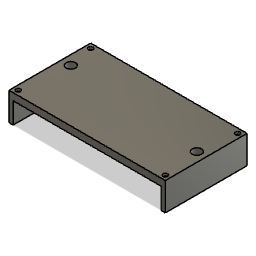
Device (Autodesk Fusion 360 archive; units mm, degrees)
design "button_holder"
Autodesk Fusion 360 part; units mm, degrees
(part 1 of 3)
sketch "Sketch1" plane through (0, 0, 0) normal (0, 1, 0) x (1, 0, 0)
  line L0 (33.5, 17.5) -> (-33.5, 17.5)
  line L1 (-33.5, 17.5) -> (-33.5, -17.5)
  line L2 (-33.5, -17.5) -> (33.5, -17.5)
  line L3 (33.5, -17.5) -> (33.5, 17.5)
  line L4 (33.5, 17.5) -> (-33.5, -17.5) construction
  line L5 (-33.5, 17.5) -> (33.5, -17.5) construction
  dimension "d1" = 67
  dimension "d2" = 35
  constraint horizontal L0
  constraint perpendicular L0 L1
  constraint parallel L0 L2
  constraint parallel L1 L3
  constraint coincident L4 origin
  constraint coincident L5 origin
  measures "d1" distance of L1.end L2.end
  measures "d2" distance of L0.end L1.end
extrude "Extrude1" add sketch "Sketch1" along normal blind 3
sketch "Sketch2" plane through (0, 0, 0) normal (0, -1, 0) x (1, 0, 0)
  line L0 (33.5, -17.5) -> (33.5, 17.5)
  line L1 (33.5, 17.5) -> (-33.5, 17.5)
  line L2 (-33.5, 17.5) -> (-33.5, -17.5)
  line L3 (-33.5, -17.5) -> (33.5, -17.5)
  line L4 (-33.5, 17.5) -> (-31.7, 17.5)
  line L5 (-31.7, 17.5) -> (-31.7, -17.5)
  line L6 (-31.7, -17.5) -> (-33.5, -17.5)
  line L7 (-33.5, -17.5) -> (-33.5, 17.5)
  line L8 (33.5, 17.5) -> (31.7, 17.5)
  line L9 (31.7, 17.5) -> (31.7, -17.5)
  line L10 (31.7, -17.5) -> (33.5, -17.5)
  line L11 (33.5, -17.5) -> (33.5, 17.5)
  dimension "d5" = 1.8
  dimension "d6" = 35
  dimension "d7" = 1.8
  dimension "d8" = 35
  constraint horizontal L4
  constraint vertical L5
  constraint horizontal L6
  constraint vertical L7
  constraint coincident L1.end L2.start
  constraint horizontal L8
  constraint vertical L9
  constraint horizontal L10
  constraint vertical L11
  constraint coincident L0.end L1.start
  measures "d5" distance of L1.end L4.end
  measures "d6" distance of L1.end L2.end
  measures "d7" distance of L0.end L8.end
  measures "d8" distance of L0.end L0.start
extrude "Extrude2" add sketch "Sketch2" along normal blind 9 contours L0 L1 L3 L8 L9 L10 L11 | L1 L2 L3 L4 L5 L6 L7
sketch "Sketch3" plane through (0, 3, 0) normal (0, 1, 0) x (-1, 0, 0)
  line L0 (-33.5, 17.5) -> (-33.5, -17.5)
  line L1 (-33.5, -17.5) -> (33.5, -17.5)
  line L2 (33.5, -17.5) -> (33.5, 17.5)
  line L3 (33.5, 17.5) -> (-33.5, 17.5)
  line L4 (33.5, -17.5) -> (31.5, -17.5)
  line L5 (31.5, -17.5) -> (31.5, -15.5)
  line L6 (31.5, -15.5) -> (33.5, -15.5)
  line L7 (33.5, -15.5) -> (33.5, -17.5)
  line L8 (33.5, 17.5) -> (31.5, 17.5)
  line L9 (31.5, 17.5) -> (31.5, 15.5)
  line L10 (31.5, 15.5) -> (33.5, 15.5)
  line L11 (33.5, 15.5) -> (33.5, 17.5)
  line L12 (-33.5, -17.5) -> (-31.5, -17.5)
  line L13 (-31.5, -17.5) -> (-31.5, -15.5)
  line L14 (-31.5, -15.5) -> (-33.5, -15.5)
  line L15 (-33.5, -15.5) -> (-33.5, -17.5)
  line L16 (-33.5, 17.5) -> (-31.5, 17.5)
  line L17 (-31.5, 17.5) -> (-31.5, 15.5)
  line L18 (-31.5, 15.5) -> (-33.5, 15.5)
  line L19 (-33.5, 15.5) -> (-33.5, 17.5)
  circle A0 centre (-31.5, 15.5) radius 1
  circle A1 centre (-31.5, -15.5) radius 1
  circle A2 centre (31.5, -15.5) radius 1
  circle A3 centre (31.5, 15.5) radius 1
  dimension "d11" = 2
  dimension "d12" = 2
  dimension "d13" = 2
  dimension "d14" = 2
  dimension "d15" = 2
  dimension "d16" = 2
  dimension "d17" = 2
  dimension "d18" = 2
  dimension "d19" = 2
  dimension "d20" = 2
  dimension "d21" = 2
  dimension "d24" = 2
  constraint horizontal L4
  constraint vertical L5
  constraint horizontal L6
  constraint vertical L7
  constraint coincident L1.end L2.start
  constraint horizontal L8
  constraint vertical L9
  constraint horizontal L10
  constraint vertical L11
  constraint coincident L2.end L3.start
  constraint horizontal L12
  constraint vertical L13
  constraint horizontal L14
  constraint vertical L15
  constraint coincident L0.end L1.start
  constraint horizontal L16
  constraint vertical L17
  constraint horizontal L18
  constraint vertical L19
  constraint coincident L0.start L3.end
  constraint coincident L17.end L18.start
  constraint coincident L13.end L14.start
  constraint coincident L5.end L6.start
  constraint coincident L9.end L10.start
  measures "d11" distance of L1.end L4.end
  measures "d12" distance of L2.end L8.end
  measures "d13" distance of L2.end L10.end
  measures "d14" distance of L0.end L12.end
  measures "d15" distance of L0.end L14.end
  measures "d16" distance of L0.start L16.end
  measures "d17" distance of L0.start L18.end
  measures "d18" diameter of A0
  measures "d19" diameter of A1
  measures "d20" diameter of A2
  measures "d21" diameter of A3
  measures "d24" distance of L1.end L6.end
extrude "Extrude3" cut sketch "Sketch3" against normal blind 1 contours L17 L18 A0 | L17 L18 A0 | L13 L14 A1 | L13 L14 A1 | L9 L10 A3 | L9 L10 A3 | L5 L6 A2 | L5 L6 A2
sketch "Sketch4" plane through (0, 3, 0) normal (0, 1, 0) x (-1, 0, 0)
  circle A0 centre (31.5, -15.5) radius 1
  circle A1 centre (-31.5, -15.5) radius 1
  circle A2 centre (31.5, 15.5) radius 1
  circle A3 centre (-31.5, 15.5) radius 1
  line L0 (-33.5, 17.5) -> (-33.5, -17.5)
  line L1 (-33.5, -17.5) -> (33.5, -17.5)
  line L2 (33.5, -17.5) -> (33.5, 17.5)
  line L3 (33.5, 17.5) -> (-33.5, 17.5)
  line L4 (-33.5, 0) -> (-29.5, 0)
  line L5 (-29.5, 0) -> (-29.5, -1)
  line L6 (-29.5, -1) -> (-33.5, -1)
  line L7 (-33.5, -1) -> (-33.5, 0)
  circle A4 centre (-29.5, 0) radius 2
  line L8 (33.5, 0) -> (29.5, 0)
  line L9 (29.5, 0) -> (29.5, -5)
  line L10 (29.5, -5) -> (33.5, -5)
  line L11 (33.5, -5) -> (33.5, 0)
  circle A5 centre (29.5, -5) radius 2
  dimension "d27" = 4
  dimension "d28" = 1
  dimension "d29" = 4
  dimension "d33" = 4
  dimension "d34" = 5
  dimension "d35" = 4
  constraint horizontal L4
  constraint vertical L5
  constraint horizontal L6
  constraint vertical L7
  constraint midpoint L0 L4.start
  constraint coincident L4.end L5.start
  constraint horizontal L8
  constraint vertical L9
  constraint horizontal L10
  constraint vertical L11
  constraint midpoint L2 L8.start
  constraint coincident L9.end L10.start
  measures "d27" distance of L4.start L4.end
  measures "d28" distance of L4.start L6.end
  measures "d29" diameter of A4
  measures "d33" distance of L8.start L8.end
  measures "d34" distance of L8.start L10.end
  measures "d35" diameter of A5
extrude "Extrude4" cut sketch "Sketch4" against normal blind 5 contours L4 L5 L6 A4 | L4 L5 L6 A4 | L9 L10 A5 | L9 L10 A5

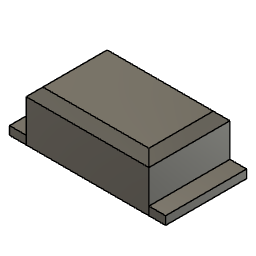
design "klavesa"
Autodesk Fusion 360 part; units mm, degrees
sketch "Sketch1" plane through (0, 0, 0) normal (0, 1, 0) x (1, 0, 0)
  line L0 (7.35, 4.85) -> (-7.35, 4.85)
  line L1 (-7.35, 4.85) -> (-7.35, -4.85)
  line L2 (-7.35, -4.85) -> (7.35, -4.85)
  line L3 (7.35, -4.85) -> (7.35, 4.85)
  line L4 (7.35, 4.85) -> (-7.35, -4.85) construction
  line L5 (-7.35, 4.85) -> (7.35, -4.85) construction
  line L6 (-7.35, 4.85) -> (-9.35, 4.85)
  line L7 (-9.35, 4.85) -> (-9.35, -4.85)
  line L8 (-9.35, -4.85) -> (-7.35, -4.85)
  line L9 (-7.35, -4.85) -> (-7.35, 4.85)
  line L10 (7.35, 4.85) -> (9.35, 4.85)
  line L11 (9.35, 4.85) -> (9.35, -4.85)
  line L12 (9.35, -4.85) -> (7.35, -4.85)
  line L13 (7.35, -4.85) -> (7.35, 4.85)
  dimension "d1" = 14.7
  dimension "d2" = 9.7
  dimension "d10" = 2
  dimension "d11" = 9.7
  dimension "d12" = 2
  dimension "d13" = 9.7
  constraint horizontal L0
  constraint perpendicular L0 L1
  constraint parallel L0 L2
  constraint parallel L1 L3
  constraint coincident L4 origin
  constraint coincident L5 origin
  constraint horizontal L6
  constraint vertical L7
  constraint horizontal L8
  constraint vertical L9
  constraint horizontal L10
  constraint vertical L11
  constraint horizontal L12
  constraint vertical L13
  measures "d1" distance of L1.end L2.end
  measures "d2" distance of L0.end L1.end
  measures "d10" distance of L0.end L6.end
  measures "d11" distance of L0.end L1.end
  measures "d12" distance of L0.start L10.end
  measures "d13" distance of L0.start L2.end
extrude "Extrude3" add sketch "Sketch1" along normal blind 1 contours L3 L10 L11 L12 L13 | L1 L6 L7 L8 L9 makes body 1 at (8.6833, 0, 1.6167) makes body 2 at (-8.0167, 0, -1.6167)
extrude "Extrude1" add sketch "Sketch1" along normal blind 6 separate body contours L0 L1 L2 L3 L9 L13 makes body 3
chamfer "Chamfer1" distance 1 angle 45 4 edges at (0, 6, 4.85) (7.35, 6, 0) (-7.35, 6, 0) (0, 6, -4.85) measured on face at (-2.45, 6, 1.6167) measured on face at (-2.45, 6, 1.6167) measured on face at (-2.45, 6, 1.6167) measured on face at (-2.45, 6, 1.6167) on bodies 3
sketch "Sketch2" plane through (0, 0, 0) normal (0, -1, 0) x (1, 0, 0)
  line L0 (7.35, -4.85) -> (7.35, 4.85)
  line L1 (7.35, 4.85) -> (-7.35, 4.85)
  line L2 (-7.35, 4.85) -> (-7.35, -4.85)
  line L3 (-7.35, -4.85) -> (7.35, -4.85)
  circle A0 centre (0, 0) radius 1.7
  dimension "d7" = 3.4
  constraint coincident A0.centre origin
  measures "d7" diameter of A0
extrude "Extrude2" cut sketch "Sketch2" against normal blind 4 contours A0 bodies 3

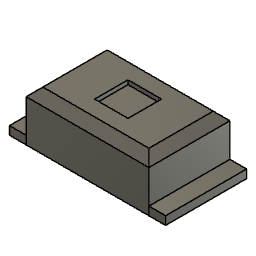
design "klavesa_stop"
Autodesk Fusion 360 part; units mm, degrees
sketch "Sketch1" plane through (0, 0, 0) normal (0, 1, 0) x (1, 0, 0)
  line L0 (7.35, 4.85) -> (-7.35, 4.85)
  line L1 (-7.35, 4.85) -> (-7.35, -4.85)
  line L2 (-7.35, -4.85) -> (7.35, -4.85)
  line L3 (7.35, -4.85) -> (7.35, 4.85)
  line L4 (7.35, 4.85) -> (-7.35, -4.85) construction
  line L5 (-7.35, 4.85) -> (7.35, -4.85) construction
  line L6 (-7.35, 4.85) -> (-9.35, 4.85)
  line L7 (-9.35, 4.85) -> (-9.35, -4.85)
  line L8 (-9.35, -4.85) -> (-7.35, -4.85)
  line L9 (-7.35, -4.85) -> (-7.35, 4.85)
  line L10 (7.35, 4.85) -> (9.35, 4.85)
  line L11 (9.35, 4.85) -> (9.35, -4.85)
  line L12 (9.35, -4.85) -> (7.35, -4.85)
  line L13 (7.35, -4.85) -> (7.35, 4.85)
  dimension "d1" = 14.7
  dimension "d2" = 9.7
  dimension "d10" = 2
  dimension "d11" = 9.7
  dimension "d12" = 2
  dimension "d13" = 9.7
  constraint horizontal L0
  constraint perpendicular L0 L1
  constraint parallel L0 L2
  constraint parallel L1 L3
  constraint coincident L4 origin
  constraint coincident L5 origin
  constraint horizontal L6
  constraint vertical L7
  constraint horizontal L8
  constraint vertical L9
  constraint horizontal L10
  constraint vertical L11
  constraint horizontal L12
  constraint vertical L13
  measures "d1" distance of L1.end L2.end
  measures "d2" distance of L0.end L1.end
  measures "d10" distance of L0.end L6.end
  measures "d11" distance of L0.end L1.end
  measures "d12" distance of L0.start L10.end
  measures "d13" distance of L0.start L2.end
extrude "Extrude3" add sketch "Sketch1" along normal blind 1 contours L3 L10 L11 L12 L13 | L1 L6 L7 L8 L9 makes body 1 at (8.6833, 0, 1.6167) makes body 2 at (-8.0167, 0, -1.6167)
extrude "Extrude1" add sketch "Sketch1" along normal blind 6 separate body contours L0 L1 L2 L3 L9 L13 makes body 3
chamfer "Chamfer1" distance 1 angle 45 4 edges at (0, 6, 4.85) (7.35, 6, 0) (-7.35, 6, 0) (0, 6, -4.85) measured on face at (-2.45, 6, 1.6167) measured on face at (-2.45, 6, 1.6167) measured on face at (-2.45, 6, 1.6167) measured on face at (-2.45, 6, 1.6167) on bodies 3
sketch "Sketch2" plane through (0, 0, 0) normal (0, -1, 0) x (1, 0, 0)
  line L0 (7.35, -4.85) -> (7.35, 4.85)
  line L1 (7.35, 4.85) -> (-7.35, 4.85)
  line L2 (-7.35, 4.85) -> (-7.35, -4.85)
  line L3 (-7.35, -4.85) -> (7.35, -4.85)
  circle A0 centre (0, 0) radius 1.7
  dimension "d7" = 3.4
  constraint coincident A0.centre origin
  measures "d7" diameter of A0
extrude "Extrude2" cut sketch "Sketch2" against normal blind 4 contours A0 bodies 3
sketch "Sketch3" plane through (0, 6, 0) normal (0, 1, 0) x (-1, 0, 0)
  line L0 (-6.35, -3.85) -> (6.35, -3.85)
  line L1 (6.35, -3.85) -> (6.35, 3.85)
  line L2 (6.35, 3.85) -> (-6.35, 3.85)
  line L3 (-6.35, 3.85) -> (-6.35, -3.85)
  line L4 (-2, -2) -> (2, -2)
  line L5 (2, -2) -> (2, 2)
  line L6 (2, 2) -> (-2, 2)
  line L7 (-2, 2) -> (-2, -2)
  line L8 (-2, -2) -> (2, 2) construction
  line L9 (2, -2) -> (-2, 2) construction
  dimension "d16" = 4
  dimension "d17" = 4
  constraint horizontal L4
  constraint perpendicular L4 L5
  constraint parallel L4 L6
  constraint parallel L5 L7
  constraint coincident L8 origin
  constraint coincident L9 origin
  measures "d16" distance of L5.end L6.end
  measures "d17" distance of L4.end L5.end
extrude "Extrude4" cut sketch "Sketch3" against normal blind 0.5 contours L4 L5 L6 L7 bodies 3

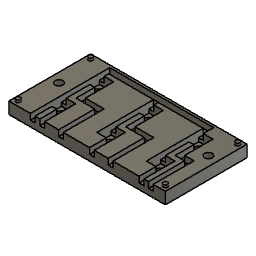
design "key_holder"
Autodesk Fusion 360 part; units mm, degrees
sketch "Sketch1" plane through (0, 0, 0) normal (0, 1, 0) x (1, 0, 0)
  line L0 (33.5, 17.5) -> (-33.5, 17.5)
  line L1 (-33.5, 17.5) -> (-33.5, -17.5)
  line L2 (-33.5, -17.5) -> (33.5, -17.5)
  line L3 (33.5, -17.5) -> (33.5, 17.5)
  line L4 (33.5, 17.5) -> (-33.5, -17.5) construction
  line L5 (-33.5, 17.5) -> (33.5, -17.5) construction
  dimension "d1" = 67
  dimension "d2" = 35
  constraint horizontal L0
  constraint perpendicular L0 L1
  constraint parallel L0 L2
  constraint parallel L1 L3
  constraint coincident L4 origin
  constraint coincident L5 origin
  measures "d1" distance of L1.end L2.end
  measures "d2" distance of L0.end L1.end
extrude "Extrude1" add sketch "Sketch1" along normal blind 5
sketch "Sketch2" plane through (0, 5, 0) normal (0, 1, 0) x (-1, 0, 0)
  line L0 (-33.5, 17.5) -> (-33.5, -17.5)
  line L1 (-33.5, -17.5) -> (33.5, -17.5)
  line L2 (33.5, -17.5) -> (33.5, 17.5)
  line L3 (33.5, 17.5) -> (-33.5, 17.5)
  line L4 (33.5, -17.5) -> (31.5, -17.5)
  line L5 (31.5, -17.5) -> (31.5, -15.5)
  line L6 (31.5, -15.5) -> (33.5, -15.5)
  line L7 (33.5, -15.5) -> (33.5, -17.5)
  line L8 (-33.5, -17.5) -> (-31.5, -17.5)
  line L9 (-31.5, -17.5) -> (-31.5, -15.5)
  line L10 (-31.5, -15.5) -> (-33.5, -15.5)
  line L11 (-33.5, -15.5) -> (-33.5, -17.5)
  line L12 (33.5, 17.5) -> (31.5, 17.5)
  line L13 (31.5, 17.5) -> (31.5, 15.5)
  line L14 (31.5, 15.5) -> (33.5, 15.5)
  line L15 (33.5, 15.5) -> (33.5, 17.5)
  line L16 (-33.5, 17.5) -> (-31.5, 17.5)
  line L17 (-31.5, 17.5) -> (-31.5, 15.5)
  line L18 (-31.5, 15.5) -> (-33.5, 15.5)
  line L19 (-33.5, 15.5) -> (-33.5, 17.5)
  circle A0 centre (-31.5, 15.5) radius 0.95
  circle A1 centre (-31.5, -15.5) radius 0.95
  circle A2 centre (31.5, -15.5) radius 0.95
  circle A3 centre (31.5, 15.5) radius 0.95
  dimension "d5" = 2
  dimension "d6" = 2
  dimension "d7" = 2
  dimension "d8" = 2
  dimension "d9" = 2
  dimension "d10" = 2
  dimension "d11" = 2
  dimension "d12" = 2
  dimension "d13" = 1.9
  dimension "d14" = 1.9
  dimension "d15" = 1.9
  dimension "d16" = 1.9
  constraint horizontal L4
  constraint vertical L5
  constraint horizontal L6
  constraint vertical L7
  constraint coincident L1.end L2.start
  constraint horizontal L8
  constraint vertical L9
  constraint horizontal L10
  constraint vertical L11
  constraint coincident L0.end L1.start
  constraint horizontal L12
  constraint vertical L13
  constraint horizontal L14
  constraint vertical L15
  constraint coincident L2.end L3.start
  constraint horizontal L16
  constraint vertical L17
  constraint horizontal L18
  constraint vertical L19
  constraint coincident L0.start L3.end
  constraint coincident L17.end L18.start
  constraint coincident L9.end L10.start
  constraint coincident L5.end L6.start
  constraint coincident L13.end L14.start
  measures "d5" distance of L1.end L4.end
  measures "d6" distance of L1.end L6.end
  measures "d7" distance of L0.end L8.end
  measures "d8" distance of L0.end L10.end
  measures "d9" distance of L2.end L12.end
  measures "d10" distance of L2.end L14.end
  measures "d11" distance of L0.start L16.end
  measures "d12" distance of L0.start L18.end
  measures "d13" diameter of A0
  measures "d14" diameter of A1
  measures "d15" diameter of A2
  measures "d16" diameter of A3
extrude "Extrude2" add sketch "Sketch2" along normal blind 1 contours L17 L18 A0 | L17 L18 A0 | L9 L10 A1 | L9 L10 A1 | L13 L14 A3 | L13 L14 A3 | L5 L6 A2 | L5 L6 A2
sketch "Sketch3" plane through (0, 5, 0) normal (0, 1, 0) x (-1, 0, 0)
  circle A0 centre (-31.5, 15.5) radius 0.95
  circle A1 centre (31.5, 15.5) radius 0.95
  circle A2 centre (-31.5, -15.5) radius 0.95
  circle A3 centre (31.5, -15.5) radius 0.95
  line L0 (-33.5, 17.5) -> (-33.5, -17.5)
  line L1 (-33.5, -17.5) -> (33.5, -17.5)
  line L2 (33.5, -17.5) -> (33.5, 17.5)
  line L3 (33.5, 17.5) -> (-33.5, 17.5)
  line L4 (33.5, -17.5) -> (28.75, -17.5)
  line L5 (28.75, -17.5) -> (28.75, -14)
  line L6 (28.75, -14) -> (33.5, -14)
  line L7 (33.5, -14) -> (33.5, -17.5)
  line L8 (28.75, -14) -> (13.75, -14)
  line L9 (13.75, -14) -> (13.75, -4)
  line L10 (13.75, -4) -> (28.75, -4)
  line L11 (28.75, -4) -> (28.75, -14)
  line L12 (13.75, -14) -> (7.5, -14)
  line L13 (7.5, -14) -> (7.5, -17.5)
  line L14 (7.5, -17.5) -> (13.75, -17.5)
  line L15 (13.75, -17.5) -> (13.75, -14)
  line L16 (7.5, -14) -> (-7.5, -14)
  line L17 (-7.5, -14) -> (-7.5, -4)
  line L18 (-7.5, -4) -> (7.5, -4)
  line L19 (7.5, -4) -> (7.5, -14)
  line L20 (-7.5, -14) -> (-13.75, -14)
  line L21 (-13.75, -14) -> (-13.75, -17.5)
  line L22 (-13.75, -17.5) -> (-7.5, -17.5)
  line L23 (-7.5, -17.5) -> (-7.5, -14)
  line L24 (-13.75, -14) -> (-28.75, -14)
  line L25 (-28.75, -14) -> (-28.75, -4)
  line L26 (-28.75, -4) -> (-13.75, -4)
  line L27 (-13.75, -4) -> (-13.75, -14)
  line L28 (-28.75, -14) -> (-33.5, -14)
  line L29 (-33.5, -14) -> (-33.5, -17.5)
  line L30 (-33.5, -17.5) -> (-28.75, -17.5)
  line L31 (-28.75, -17.5) -> (-28.75, -14)
  line L32 (28.75, -4) -> (33.5, -4)
  line L33 (33.5, -4) -> (33.5, 2.25)
  line L34 (33.5, 2.25) -> (28.75, 2.25)
  line L35 (28.75, 2.25) -> (28.75, -4)
  line L36 (28.75, 2.25) -> (13.75, 2.25)
  line L37 (13.75, 2.25) -> (13.75, 12.25)
  line L38 (13.75, 12.25) -> (28.75, 12.25)
  line L39 (28.75, 12.25) -> (28.75, 2.25)
  line L40 (13.75, 2.25) -> (7.5, 2.25)
  line L41 (7.5, 2.25) -> (7.5, -4)
  line L42 (7.5, -4) -> (13.75, -4)
  line L43 (13.75, -4) -> (13.75, 2.25)
  line L44 (7.5, 2.25) -> (-7.5, 2.25)
  line L45 (-7.5, 2.25) -> (-7.5, 12.25)
  line L46 (-7.5, 12.25) -> (7.5, 12.25)
  line L47 (7.5, 12.25) -> (7.5, 2.25)
  line L48 (-7.5, 2.25) -> (-13.75, 2.25)
  line L49 (-13.75, 2.25) -> (-13.75, -4)
  line L50 (-13.75, -4) -> (-7.5, -4)
  line L51 (-7.5, -4) -> (-7.5, 2.25)
  line L52 (-13.75, 2.25) -> (-28.75, 2.25)
  line L53 (-28.75, 2.25) -> (-28.75, 12.25)
  line L54 (-28.75, 12.25) -> (-13.75, 12.25)
  line L55 (-13.75, 12.25) -> (-13.75, 2.25)
  line L56 (-13.75, 12.25) -> (-28.75, 2.25)
  line L57 (-13.75, 2.25) -> (-28.75, 12.25)
  line L58 (-13.75, -4) -> (-28.75, -14)
  line L59 (-13.75, -14) -> (-28.75, -4)
  line L60 (7.5, -14) -> (-7.5, -4)
  line L61 (7.5, -4) -> (-7.5, -14)
  line L62 (7.5, 2.25) -> (-7.5, 12.25)
  line L63 (7.5, 12.25) -> (-7.5, 2.25)
  line L64 (13.75, 12.25) -> (28.75, 2.25)
  line L65 (28.75, 12.25) -> (13.75, 2.25)
  line L66 (28.75, -4) -> (13.75, -14)
  line L67 (28.75, -14) -> (13.75, -4)
  line L68 (18.2, -12.05) -> (24.3, -12.05)
  line L69 (24.3, -12.05) -> (24.3, -5.95)
  line L70 (24.3, -5.95) -> (18.2, -5.95)
  line L71 (18.2, -5.95) -> (18.2, -12.05)
  line L72 (18.2, -12.05) -> (24.3, -5.95) construction
  line L73 (24.3, -12.05) -> (18.2, -5.95) construction
  line L74 (-3.05, -12.05) -> (3.05, -12.05)
  line L75 (3.05, -12.05) -> (3.05, -5.95)
  line L76 (3.05, -5.95) -> (-3.05, -5.95)
  line L77 (-3.05, -5.95) -> (-3.05, -12.05)
  line L78 (-3.05, -12.05) -> (3.05, -5.95) construction
  line L79 (3.05, -12.05) -> (-3.05, -5.95) construction
  line L80 (-24.3, -12.05) -> (-18.2, -12.05)
  line L81 (-18.2, -12.05) -> (-18.2, -5.95)
  line L82 (-18.2, -5.95) -> (-24.3, -5.95)
  line L83 (-24.3, -5.95) -> (-24.3, -12.05)
  line L84 (-24.3, -12.05) -> (-18.2, -5.95) construction
  line L85 (-18.2, -12.05) -> (-24.3, -5.95) construction
  line L86 (-24.3, 4.2) -> (-18.2, 4.2)
  line L87 (-18.2, 4.2) -> (-18.2, 10.3)
  line L88 (-18.2, 10.3) -> (-24.3, 10.3)
  line L89 (-24.3, 10.3) -> (-24.3, 4.2)
  line L90 (-24.3, 4.2) -> (-18.2, 10.3) construction
  line L91 (-18.2, 4.2) -> (-24.3, 10.3) construction
  line L92 (-3.05, 4.2) -> (3.05, 4.2)
  line L93 (3.05, 4.2) -> (3.05, 10.3)
  line L94 (3.05, 10.3) -> (-3.05, 10.3)
  line L95 (-3.05, 10.3) -> (-3.05, 4.2)
  line L96 (-3.05, 4.2) -> (3.05, 10.3) construction
  line L97 (3.05, 4.2) -> (-3.05, 10.3) construction
  line L98 (18.2, 4.2) -> (24.3, 4.2)
  line L99 (24.3, 4.2) -> (24.3, 10.3)
  line L100 (24.3, 10.3) -> (18.2, 10.3)
  line L101 (18.2, 10.3) -> (18.2, 4.2)
  line L102 (18.2, 4.2) -> (24.3, 10.3) construction
  line L103 (24.3, 4.2) -> (18.2, 10.3) construction
  circle A4 centre (21.25, -9) radius 2
  circle A5 centre (0, -9) radius 2
  circle A6 centre (-21.25, -9) radius 2
  circle A7 centre (21.25, 7.25) radius 2
  circle A8 centre (0, 7.25) radius 2
  circle A9 centre (-21.25, 7.25) radius 2
  point P0 (21.25, -9)
  point P1 (0, -9)
  point P2 (-21.25, -9)
  point P3 (-21.25, 7.25)
  point P4 (0, 7.25)
  point P5 (21.25, 7.25)
  dimension "d19" = 4.75
  dimension "d20" = 3.5
  dimension "d21" = 15
  dimension "d22" = 10
  dimension "d23" = 6.25
  dimension "d24" = 15
  dimension "d25" = 10
  dimension "d26" = 6.25
  dimension "d27" = 15
  dimension "d28" = 10
  dimension "d29" = 4.75
  dimension "d30" = 3.5
  dimension "d31" = 6.25
  dimension "d32" = 15
  dimension "d33" = 10
  dimension "d34" = 6.25
  dimension "d35" = 6.25
  dimension "d36" = 15
  dimension "d37" = 10
  dimension "d38" = 6.25
  dimension "d39" = 6.25
  dimension "d40" = 15
  dimension "d41" = 10
  dimension "d42" = 6.1
  dimension "d43" = 6.1
  dimension "d44" = 6.1
  dimension "d45" = 6.1
  dimension "d46" = 6.1
  dimension "d47" = 6.1
  dimension "d48" = 6.1
  dimension "d49" = 6.1
  dimension "d50" = 6.1
  dimension "d51" = 6.1
  dimension "d52" = 6.1
  dimension "d53" = 6.1
  dimension "d56" = 4
  dimension "d57" = 4
  dimension "d58" = 4
  dimension "d59" = 4
  dimension "d60" = 4
  dimension "d61" = 4
  constraint horizontal L4
  constraint vertical L5
  constraint horizontal L6
  constraint vertical L7
  constraint coincident L1.end L2.start
  constraint horizontal L8
  constraint vertical L9
  constraint horizontal L10
  constraint vertical L11
  constraint horizontal L12
  constraint vertical L13
  constraint horizontal L14
  constraint vertical L15
  constraint horizontal L16
  constraint vertical L17
  constraint horizontal L18
  constraint vertical L19
  constraint horizontal L20
  constraint vertical L21
  constraint horizontal L22
  constraint vertical L23
  constraint horizontal L24
  constraint vertical L25
  constraint horizontal L26
  constraint vertical L27
  constraint horizontal L28
  constraint vertical L29
  constraint horizontal L30
  constraint vertical L31
  constraint horizontal L32
  constraint vertical L33
  constraint horizontal L34
  constraint vertical L35
  constraint horizontal L36
  constraint vertical L37
  constraint horizontal L38
  constraint vertical L39
  constraint horizontal L40
  constraint vertical L41
  constraint horizontal L42
  constraint vertical L43
  constraint horizontal L44
  constraint vertical L45
  constraint horizontal L46
  constraint vertical L47
  constraint horizontal L48
  constraint vertical L49
  constraint horizontal L50
  constraint vertical L51
  constraint horizontal L52
  constraint vertical L53
  constraint horizontal L54
  constraint vertical L55
  constraint horizontal L68
  constraint perpendicular L68 L69
  constraint parallel L68 L70
  constraint parallel L69 L71
  constraint coincident L72 P0
  constraint coincident L73 P0
  constraint midpoint L67 P0
  constraint horizontal L74
  constraint perpendicular L74 L75
  constraint parallel L74 L76
  constraint parallel L75 L77
  constraint coincident L78 P1
  constraint coincident L79 P1
  constraint midpoint L60 P1
  constraint horizontal L80
  constraint perpendicular L80 L81
  constraint parallel L80 L82
  constraint parallel L81 L83
  constraint coincident L84 P2
  constraint coincident L85 P2
  constraint midpoint L59 P2
  constraint horizontal L86
  constraint perpendicular L86 L87
  constraint parallel L86 L88
  constraint parallel L87 L89
  constraint coincident L90 P3
  constraint coincident L91 P3
  constraint midpoint L56 P3
  constraint horizontal L92
  constraint perpendicular L92 L93
  constraint parallel L92 L94
  constraint parallel L93 L95
  constraint coincident L96 P4
  constraint coincident L97 P4
  constraint midpoint L62 P4
  constraint horizontal L98
  constraint perpendicular L98 L99
  constraint parallel L98 L100
  constraint parallel L99 L101
  constraint coincident L102 P5
  constraint coincident L103 P5
  constraint midpoint L64 P5
  constraint coincident P0 A4.centre
  constraint coincident P1 A5.centre
  constraint coincident P2 A6.centre
  constraint coincident P5 A7.centre
  constraint coincident P4 A8.centre
  constraint coincident P3 A9.centre
  measures "d19" distance of L1.end L4.end
  measures "d20" distance of L1.end L6.end
  measures "d21" distance of L5.end L8.end
  measures "d22" distance of L5.end L10.end
  measures "d23" distance of L8.end L12.end
  measures "d24" distance of L12.end L16.end
  measures "d25" distance of L12.end L18.end
  measures "d26" distance of L16.end L20.end
  measures "d27" distance of L20.end L24.end
  measures "d28" distance of L20.end L26.end
  measures "d29" distance of L24.end L28.end
  measures "d30" distance of L24.end L30.end
  measures "d31" distance of L10.end L34.end
  measures "d32" distance of L34.end L36.end
  measures "d33" distance of L34.end L38.end
  measures "d34" distance of L36.end L40.end
  measures "d35" distance of L36.end L9.end
  measures "d36" distance of L40.end L44.end
  measures "d37" distance of L40.end L46.end
  measures "d38" distance of L44.end L48.end
  measures "d39" distance of L44.end L17.end
  measures "d40" distance of L48.end L52.end
  measures "d41" distance of L48.end L54.end
  measures "d42" distance of L69.end L70.end
  measures "d43" distance of L68.end L69.end
  measures "d44" distance of L75.end L76.end
  measures "d45" distance of L74.end L75.end
  measures "d46" distance of L81.end L82.end
  measures "d47" distance of L80.end L81.end
  measures "d48" distance of L87.end L88.end
  measures "d49" distance of L86.end L87.end
  measures "d50" distance of L93.end L94.end
  measures "d51" distance of L92.end L93.end
  measures "d52" distance of L99.end L100.end
  measures "d53" distance of L98.end L99.end
  measures "d56" diameter of A4
  measures "d57" diameter of A5
  measures "d58" diameter of A6
  measures "d59" diameter of A7
  measures "d60" diameter of A8
  measures "d61" diameter of A9
extrude "Extrude4" cut sketch "Sketch3" against normal blind 6 contours L58 L59 A6 | L58 L59 A6 | L58 L59 A6 | L58 L59 A6 | L64 L65 A7 | L64 L65 A7 | L60 L61 A5 | L60 L61 A5 | L66 L67 A4 | L66 L67 A4 | L64 L65 A7 | L64 L65 A7 | L60 L61 A5 | L60 L61 A5 | L56 L57 A9 | L56 L57 A9 | L66 L67 A4 | L66 L67 A4 | L62 L63 A8 | L62 L63 A8 | L62 L63 A8 | L56 L57 A9 | L56 L57 A9 | L62 L63 A8
extrude "Extrude3" cut sketch "Sketch3" against normal blind 4 contours L58 L59 L83 A6 | L58 L59 L80 L81 L83 A6 | L58 L59 L81 A6 | L58 L59 L81 L82 L83 A6 | L58 L59 A6 | L58 L59 A6 | L64 L65 L98 L99 L101 A7 | L64 L65 L99 A7 | L60 L61 L77 A5 | L60 L61 L74 L75 L77 A5 | L58 L59 A6 | L58 L59 A6 | L66 L67 L69 A4 | L66 L67 L69 L70 L71 A4 | L64 L65 L101 A7 | L64 L65 L99 L100 L101 A7 | L64 L65 A7 | L64 L65 A7 | L60 L61 L75 A5 | L60 L61 L75 L76 L77 A5 | L60 L61 A5 | L60 L61 A5 | L56 L57 L86 L87 L89 A9 | L56 L57 L87 A9 | L66 L67 L68 L69 L71 A4 | L66 L67 L71 A4 | L66 L67 A4 | L66 L67 A4 | L62 L63 L92 L93 L95 A8 | L62 L63 L93 A8 | L64 L65 A7 | L64 L65 A7 | L60 L61 A5 | L62 L63 L95 A8 | L60 L61 A5 | L56 L57 L89 A9 | L56 L57 L87 L88 L89 A9 | L56 L57 A9 | L56 L57 A9 | L66 L67 A4 | L66 L67 A4 | L62 L63 L93 L94 L95 A8 | L62 L63 A8 | L62 L63 A8 | L62 L63 A8 | L56 L57 A9 | L56 L57 A9 | L62 L63 A8
sketch "Sketch4" plane through (0, 5, 0) normal (0, 1, 0) x (-1, 0, 0)
  line L0 (-18.2, 4.2) -> (-24.3, 4.2)
  line L1 (-24.3, 4.2) -> (-24.3, 10.3)
  line L2 (-24.3, 10.3) -> (-18.2, 10.3)
  line L3 (-18.2, 10.3) -> (-18.2, 4.2)
  line L4 (24.3, -12.05) -> (18.2, -12.05)
  line L5 (18.2, -12.05) -> (18.2, -5.95)
  line L6 (18.2, -5.95) -> (24.3, -5.95)
  line L7 (24.3, -5.95) -> (24.3, -12.05)
  line L8 (3.05, 4.2) -> (-3.05, 4.2)
  line L9 (-3.05, 4.2) -> (-3.05, 10.3)
  line L10 (-3.05, 10.3) -> (3.05, 10.3)
  line L11 (3.05, 10.3) -> (3.05, 4.2)
  line L12 (-18.2, -12.05) -> (-24.3, -12.05)
  line L13 (-24.3, -12.05) -> (-24.3, -5.95)
  line L14 (-24.3, -5.95) -> (-18.2, -5.95)
  line L15 (-18.2, -5.95) -> (-18.2, -12.05)
  line L16 (3.05, -12.05) -> (-3.05, -12.05)
  line L17 (-3.05, -12.05) -> (-3.05, -5.95)
  line L18 (-3.05, -5.95) -> (3.05, -5.95)
  line L19 (3.05, -5.95) -> (3.05, -12.05)
  line L20 (24.3, 4.2) -> (18.2, 4.2)
  line L21 (18.2, 4.2) -> (18.2, 10.3)
  line L22 (18.2, 10.3) -> (24.3, 10.3)
  line L23 (24.3, 10.3) -> (24.3, 4.2)
  circle A0 centre (-31.5, 15.5) radius 0.95
  circle A1 centre (31.5, 15.5) radius 0.95
  circle A2 centre (-31.5, -15.5) radius 0.95
  circle A3 centre (31.5, -15.5) radius 0.95
  line L24 (-33.5, 17.5) -> (-33.5, -17.5)
  line L25 (-33.5, -17.5) -> (33.5, -17.5)
  line L26 (33.5, -17.5) -> (33.5, 17.5)
  line L27 (33.5, 17.5) -> (-33.5, 17.5)
  line L28 (24.3, -5.95) -> (22.3, -5.95)
  line L29 (22.3, -5.95) -> (22.3, 4.2)
  line L30 (22.3, 4.2) -> (24.3, 4.2)
  line L31 (24.3, 4.2) -> (24.3, -5.95)
  line L32 (24.3, 10.3) -> (22.3, 10.3)
  line L33 (22.3, 10.3) -> (22.3, 17.5)
  line L34 (22.3, 17.5) -> (24.3, 17.5)
  line L35 (24.3, 17.5) -> (24.3, 10.3)
  line L36 (24.3, -12.05) -> (22.3, -12.05)
  line L37 (22.3, -12.05) -> (22.3, -17.5)
  line L38 (22.3, -17.5) -> (24.3, -17.5)
  line L39 (24.3, -17.5) -> (24.3, -12.05)
  line L40 (3.05, -12.05) -> (1.05, -12.05)
  line L41 (1.05, -12.05) -> (1.05, -17.5)
  line L42 (1.05, -17.5) -> (3.05, -17.5)
  line L43 (3.05, -17.5) -> (3.05, -12.05)
  line L44 (3.05, -5.95) -> (1.05, -5.95)
  line L45 (1.05, -5.95) -> (1.05, 4.2)
  line L46 (1.05, 4.2) -> (3.05, 4.2)
  line L47 (3.05, 4.2) -> (3.05, -5.95)
  line L48 (3.05, 10.3) -> (1.05, 10.3)
  line L49 (1.05, 10.3) -> (1.05, 17.5)
  line L50 (1.05, 17.5) -> (3.05, 17.5)
  line L51 (3.05, 17.5) -> (3.05, 10.3)
  line L52 (-18.2, -12.05) -> (-20.2, -12.05)
  line L53 (-20.2, -12.05) -> (-20.2, -17.5)
  line L54 (-20.2, -17.5) -> (-18.2, -17.5)
  line L55 (-18.2, -17.5) -> (-18.2, -12.05)
  line L56 (-18.2, -5.95) -> (-20.2, -5.95)
  line L57 (-20.2, -5.95) -> (-20.2, 4.2)
  line L58 (-20.2, 4.2) -> (-18.2, 4.2)
  line L59 (-18.2, 4.2) -> (-18.2, -5.95)
  line L60 (-18.2, 10.3) -> (-20.2, 10.3)
  line L61 (-20.2, 10.3) -> (-20.2, 17.5)
  line L62 (-20.2, 17.5) -> (-18.2, 17.5)
  line L63 (-18.2, 17.5) -> (-18.2, 10.3)
  line L64 (22.3, -13.9836) -> (-20.2, -13.9836)
  line L65 (-20.2, -13.9836) -> (-20.2, -16.4836)
  line L66 (-20.2, -16.4836) -> (22.3, -16.4836)
  line L67 (22.3, -16.4836) -> (22.3, -13.9836)
  line L68 (18.2, -5.95) -> (20.2, -5.95)
  line L69 (20.2, -5.95) -> (20.2, 0.05)
  line L70 (20.2, 0.05) -> (18.2, 0.05)
  line L71 (18.2, 0.05) -> (18.2, -5.95)
  line L72 (20.2, 0.05) -> (10.2, 0.05)
  line L73 (10.2, 0.05) -> (10.2, 2.05)
  line L74 (10.2, 2.05) -> (20.2, 2.05)
  line L75 (20.2, 2.05) -> (20.2, 0.05)
  line L76 (10.2, 2.05) -> (12.2, 2.05)
  line L77 (12.2, 2.05) -> (12.2, 17.5)
  line L78 (12.2, 17.5) -> (10.2, 17.5)
  line L79 (10.2, 17.5) -> (10.2, 2.05)
  line L80 (18.2, 10.3) -> (20.2, 10.3)
  line L81 (20.2, 10.3) -> (20.2, 17.5)
  line L82 (20.2, 17.5) -> (18.2, 17.5)
  line L83 (18.2, 17.5) -> (18.2, 10.3)
  line L84 (-3.05, 10.3) -> (-1.05, 10.3)
  line L85 (-1.05, 10.3) -> (-1.05, 17.5)
  line L86 (-1.05, 17.5) -> (-3.05, 17.5)
  line L87 (-3.05, 17.5) -> (-3.05, 10.3)
  line L88 (-24.3, 10.3) -> (-22.3, 10.3)
  line L89 (-22.3, 10.3) -> (-22.3, 17.5)
  line L90 (-22.3, 17.5) -> (-24.3, 17.5)
  line L91 (-24.3, 17.5) -> (-24.3, 10.3)
  line L92 (-3.05, -5.95) -> (-1.05, -5.95)
  line L93 (-1.05, -5.95) -> (-1.05, 0.05)
  line L94 (-1.05, 0.05) -> (-3.05, 0.05)
  line L95 (-3.05, 0.05) -> (-3.05, -5.95)
  line L96 (-24.3, -5.95) -> (-22.3, -5.95)
  line L97 (-22.3, -5.95) -> (-22.3, 0.05)
  line L98 (-22.3, 0.05) -> (-24.3, 0.05)
  line L99 (-24.3, 0.05) -> (-24.3, -5.95)
  line L100 (-1.05, 0.05) -> (-11.05, 0.05)
  line L101 (-11.05, 0.05) -> (-11.05, 2.05)
  line L102 (-11.05, 2.05) -> (-1.05, 2.05)
  line L103 (-1.05, 2.05) -> (-1.05, 0.05)
  line L104 (-11.05, 2.05) -> (-9.05, 2.05)
  line L105 (-9.05, 2.05) -> (-9.05, 17.5)
  line L106 (-9.05, 17.5) -> (-11.05, 17.5)
  line L107 (-11.05, 17.5) -> (-11.05, 2.05)
  line L108 (-22.3, 0.05) -> (-28.3, 0.05)
  line L109 (-28.3, 0.05) -> (-28.3, 2.05)
  line L110 (-28.3, 2.05) -> (-22.3, 2.05)
  line L111 (-22.3, 2.05) -> (-22.3, 0.05)
  line L112 (22.3, -16.4836) -> (24.3, -16.4836)
  line L113 (24.3, -16.4836) -> (24.3, -17.5)
  line L114 (24.3, -17.5) -> (22.3, -17.5)
  line L115 (22.3, -17.5) -> (22.3, -16.4836)
  line L116 (-28.3, 2.05) -> (-26.3, 2.05)
  line L117 (-26.3, 2.05) -> (-26.3, 17.5)
  line L118 (-26.3, 17.5) -> (-28.3, 17.5)
  line L119 (-28.3, 17.5) -> (-28.3, 2.05)
  dimension "d64" = 2
  dimension "d65" = 2
  dimension "d66" = 2
  dimension "d67" = 2
  dimension "d68" = 2
  dimension "d69" = 2
  dimension "d70" = 2
  dimension "d71" = 2
  dimension "d72" = 2
  dimension "d73" = 2.5
  dimension "d76" = 2
  dimension "d77" = 6
  dimension "d78" = 10
  dimension "d79" = 2
  dimension "d80" = 2
  dimension "d81" = 2
  dimension "d82" = 2
  dimension "d83" = 2
  dimension "d84" = 2
  dimension "d85" = 6
  dimension "d86" = 2
  dimension "d87" = 6
  dimension "d88" = 10
  dimension "d89" = 2
  dimension "d90" = 2
  dimension "d91" = 6
  dimension "d92" = 2
  dimension "d94" = 2
  constraint horizontal L28
  constraint vertical L29
  constraint horizontal L30
  constraint vertical L31
  constraint coincident L6.end L7.start
  constraint horizontal L32
  constraint vertical L33
  constraint horizontal L34
  constraint vertical L35
  constraint coincident L22.end L23.start
  constraint horizontal L36
  constraint vertical L37
  constraint horizontal L38
  constraint vertical L39
  constraint coincident L4.start L7.end
  constraint horizontal L40
  constraint vertical L41
  constraint horizontal L42
  constraint vertical L43
  constraint coincident L16.start L19.end
  constraint horizontal L44
  constraint vertical L45
  constraint horizontal L46
  constraint vertical L47
  constraint coincident L18.end L19.start
  constraint horizontal L48
  constraint vertical L49
  constraint horizontal L50
  constraint vertical L51
  constraint coincident L10.end L11.start
  constraint horizontal L52
  constraint vertical L53
  constraint horizontal L54
  constraint vertical L55
  constraint coincident L12.start L15.end
  constraint horizontal L56
  constraint vertical L57
  constraint horizontal L58
  constraint vertical L59
  constraint coincident L14.end L15.start
  constraint horizontal L60
  constraint vertical L61
  constraint horizontal L62
  constraint vertical L63
  constraint coincident L2.end L3.start
  constraint horizontal L64
  constraint vertical L65
  constraint horizontal L66
  constraint vertical L67
  constraint coincident L37 L64.start
  constraint horizontal L68
  constraint vertical L69
  constraint horizontal L70
  constraint vertical L71
  constraint coincident L5.end L6.start
  constraint horizontal L72
  constraint vertical L73
  constraint horizontal L74
  constraint vertical L75
  constraint horizontal L76
  constraint vertical L77
  constraint horizontal L78
  constraint vertical L79
  constraint horizontal L80
  constraint vertical L81
  constraint horizontal L82
  constraint vertical L83
  constraint coincident L21.end L22.start
  constraint horizontal L84
  constraint vertical L85
  constraint horizontal L86
  constraint vertical L87
  constraint coincident L9.end L10.start
  constraint horizontal L88
  constraint vertical L89
  constraint horizontal L90
  constraint vertical L91
  constraint coincident L1.end L2.start
  constraint horizontal L92
  constraint vertical L93
  constraint horizontal L94
  constraint vertical L95
  constraint coincident L17.end L18.start
  constraint horizontal L96
  constraint vertical L97
  constraint horizontal L98
  constraint vertical L99
  constraint coincident L13.end L14.start
  constraint horizontal L100
  constraint vertical L101
  constraint horizontal L102
  constraint vertical L103
  constraint horizontal L104
  constraint vertical L105
  constraint horizontal L106
  constraint vertical L107
  constraint horizontal L108
  constraint vertical L109
  constraint horizontal L110
  constraint vertical L111
  constraint horizontal L112
  constraint vertical L113
  constraint horizontal L114
  constraint vertical L115
  constraint horizontal L116
  constraint vertical L117
  constraint horizontal L118
  constraint vertical L119
  constraint coincident L27 L117.end
  measures "d64" distance of L6.end L28.end
  measures "d65" distance of L22.end L32.end
  measures "d66" distance of L4.start L36.end
  measures "d67" distance of L16.start L40.end
  measures "d68" distance of L18.end L44.end
  measures "d69" distance of L10.end L48.end
  measures "d70" distance of L12.start L52.end
  measures "d71" distance of L14.end L56.end
  measures "d72" distance of L2.end L60.end
  measures "d73" distance of L64.start L66.end
  measures "d76" distance of L5.end L68.end
  measures "d77" distance of L5.end L70.end
  measures "d78" distance of L69.end L72.end
  measures "d79" distance of L69.end L74.end
  measures "d80" distance of L73.end L76.end
  measures "d81" distance of L21.end L80.end
  measures "d82" distance of L9.end L84.end
  measures "d83" distance of L1.end L88.end
  measures "d84" distance of L17.end L92.end
  measures "d85" distance of L17.end L94.end
  measures "d86" distance of L13.end L96.end
  measures "d87" distance of L13.end L98.end
  measures "d88" distance of L93.end L100.end
  measures "d89" distance of L93.end L102.end
  measures "d90" distance of L101.end L104.end
  measures "d91" distance of L97.end L108.end
  measures "d92" distance of L97.end L110.end
  measures "d94" distance of L109.end L116.end
extrude "Extrude5" cut sketch "Sketch4" against normal blind 2.5 contours L0 L14 L56 L57 L58 L59 | L12 L52 L53 L55 L64 | L2 L27 L88 L89 L90 L91 | L14 L96 L97 L98 L99 L108 | L27 L102 L104 L105 L106 L107 | L41 L55 L64 L66 | L53 L55 L64 L65 L66 | L98 L108 L109 L110 L111 L116 | L94 L100 L101 L102 L103 L104 | L41 L43 L64 L66 | L16 L40 L41 L43 L64 | L27 L110 L116 L117 L118 L119 | L10 L27 L84 L85 L86 L87 | L37 L43 L64 L66 L67 | L18 L92 L93 L94 L95 L100 | L4 L36 L37 L39 L67 L112 | L8 L18 L44 L45 L46 L47 | L27 L74 L76 L77 L78 L79 | L6 L20 L28 L29 L30 L31 | L6 L68 L69 L70 L71 L72 | L70 L72 L73 L74 L75 L76 | L22 L27 L80 L81 L82 L83 | L22 L27 L32 L33 L34 L35
sketch "Sketch5" plane through (0, 5, 0) normal (0, 1, 0) x (-1, 0, 0)
  circle A0 centre (31.5, -15.5) radius 0.95
  circle A1 centre (-31.5, -15.5) radius 0.95
  circle A2 centre (31.5, 15.5) radius 0.95
  circle A3 centre (-31.5, 15.5) radius 0.95
  line L0 (24.3, 17.5) -> (24.3, -16.4836)
  line L1 (24.3, -16.4836) -> (-20.2, -16.4836)
  line L2 (-20.2, -16.4836) -> (-20.2, -12.05)
  line L3 (-20.2, -12.05) -> (-24.3, -12.05)
  line L4 (-24.3, -12.05) -> (-24.3, 0.05)
  line L5 (-24.3, 0.05) -> (-28.3, 0.05)
  line L6 (-28.3, 0.05) -> (-28.3, 17.5)
  line L7 (-28.3, 17.5) -> (-33.5, 17.5)
  line L8 (-33.5, 17.5) -> (-33.5, -17.5)
  line L9 (-33.5, -17.5) -> (33.5, -17.5)
  line L10 (33.5, -17.5) -> (33.5, 17.5)
  line L11 (33.5, 17.5) -> (24.3, 17.5)
  line L12 (33.5, 0) -> (29.5, 0)
  line L13 (29.5, 0) -> (29.5, 1)
  line L14 (29.5, 1) -> (33.5, 1)
  line L15 (33.5, 1) -> (33.5, 0)
  circle A4 centre (29.5, 0) radius 1.65
  line L16 (-33.5, 0) -> (-29.5, 0)
  line L17 (-29.5, 0) -> (-29.5, -5)
  line L18 (-29.5, -5) -> (-33.5, -5)
  line L19 (-33.5, -5) -> (-33.5, 0)
  circle A5 centre (-29.5, -5) radius 1.65
  circle A6 centre (29.5, 0) radius 2.75
  circle A7 centre (-29.5, -5) radius 2.75
  dimension "d97" = 4
  dimension "d98" = 1
  dimension "d99" = 3.3
  dimension "d102" = 3.3
  dimension "d103" = 4
  dimension "d104" = 5
  dimension "d105" = 5.5
  dimension "d106" = 5.5
  constraint horizontal L12
  constraint vertical L13
  constraint horizontal L14
  constraint vertical L15
  constraint midpoint L10 L12.start
  constraint coincident L12.end L13.start
  constraint horizontal L16
  constraint vertical L17
  constraint horizontal L18
  constraint vertical L19
  constraint midpoint L8 L16.start
  constraint coincident L17.end L18.start
  measures "d97" distance of L12.start L12.end
  measures "d98" distance of L12.start L14.end
  measures "d99" diameter of A4
  measures "d102" diameter of A5
  measures "d103" distance of L17.end L18.end
  measures "d104" distance of L16.start L18.end
  measures "d105" diameter of A6
  measures "d106" diameter of A7
extrude "Extrude6" cut sketch "Sketch5" against normal blind 6 contours L12 L13 L14 A4 | L12 L13 L14 A4 | L17 L18 A5 | L17 L18 A5
sketch "Sketch6" plane through (0, 0, 0) normal (0, -1, 0) x (1, 0, 0)
  circle A0 centre (-29.5, 0) radius 1.65
  circle A1 centre (29.5, -5) radius 1.65
  circle A2 centre (0, -9) radius 2
  circle A3 centre (21.25, 7.25) radius 2
  circle A4 centre (-21.25, -9) radius 2
  circle A5 centre (21.25, -9) radius 2
  circle A6 centre (0, 7.25) radius 2
  circle A7 centre (-21.25, 7.25) radius 2
  line L0 (33.5, -17.5) -> (33.5, 17.5)
  line L1 (33.5, 17.5) -> (-33.5, 17.5)
  line L2 (-33.5, 17.5) -> (-33.5, -17.5)
  line L3 (-33.5, -17.5) -> (33.5, -17.5)
  line L4 (-33.5, 0) -> (-29.5, 0)
  line L5 (-29.5, 0) -> (-29.5, -1)
  line L6 (-29.5, -1) -> (-33.5, -1)
  line L7 (-33.5, -1) -> (-33.5, 0)
  circle A8 centre (-29.5, 0) radius 2.75
  line L8 (33.5, 0) -> (29.5, 0)
  line L9 (29.5, 0) -> (29.5, -5)
  line L10 (29.5, -5) -> (33.5, -5)
  line L11 (33.5, -5) -> (33.5, 0)
  circle A9 centre (29.5, -5) radius 2.75
  dimension "d107" = 4
  dimension "d108" = 1
  dimension "d109" = 5.5
  dimension "d110" = 4
  dimension "d111" = 5
  dimension "d112" = 5.5
  constraint horizontal L4
  constraint vertical L5
  constraint horizontal L6
  constraint vertical L7
  constraint midpoint L2 L4.start
  constraint coincident A0.centre L4.end
  constraint horizontal L8
  constraint vertical L9
  constraint horizontal L10
  constraint vertical L11
  constraint midpoint L0 L8.start
  constraint coincident A1.centre L9.end
  measures "d107" distance of L4.start A0.centre
  measures "d108" distance of L4.start L6.end
  measures "d109" diameter of A8
  measures "d110" distance of L8.start L8.end
  measures "d111" distance of L8.start L10.end
  measures "d112" diameter of A9
extrude "Extrude7" cut sketch "Sketch6" against normal blind 2.5 contours A0 L4 L6 A8 | A0 L4 L6 A8 | A1 L9 L10 A9 | A1 L9 L10 A9

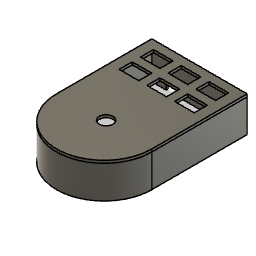
design "top"
Autodesk Fusion 360 part; units mm, degrees
sketch "Sketch1" plane through (0, 0, 0) normal (0, 1, 0) x (1, 0, 0)
  line L0 (35, 35) -> (-35, 35)
  line L1 (-35, 35) -> (-35, -35)
  line L2 (-35, -35) -> (35, -35)
  line L3 (35, -35) -> (35, 35)
  line L4 (35, 35) -> (-35, -35) construction
  line L5 (-35, 35) -> (35, -35) construction
  circle A0 centre (0, -35) radius 35
  line L6 (36.5, 36.5) -> (-36.5, 36.5)
  line L7 (-36.5, 36.5) -> (-36.5, -36.5)
  line L8 (-36.5, -36.5) -> (36.5, -36.5)
  line L9 (36.5, -36.5) -> (36.5, 36.5)
  line L10 (36.5, 36.5) -> (-36.5, -36.5) construction
  line L11 (-36.5, 36.5) -> (36.5, -36.5) construction
  circle A1 centre (0, -36.5) radius 36.5
  circle A2 centre (0, -35) radius 5.25
  dimension "d1" = 70
  dimension "d2" = 70
  dimension "d3" = 70
  dimension "d4" = 73
  dimension "d5" = 73
  dimension "d6" = 73
  dimension "d11" = 10.5
  constraint horizontal L0
  constraint perpendicular L0 L1
  constraint parallel L0 L2
  constraint parallel L1 L3
  constraint coincident L4 origin
  constraint coincident L5 origin
  constraint midpoint L2 A0.centre
  constraint horizontal L6
  constraint perpendicular L6 L7
  constraint parallel L6 L8
  constraint parallel L7 L9
  constraint coincident L10 origin
  constraint coincident L11 origin
  constraint midpoint L8 A1.centre
  constraint concentric A0 A2
  measures "d1" distance of L1.end L2.end
  measures "d2" distance of L0.end L1.end
  measures "d3" diameter of A0
  measures "d4" distance of L7.end L8.end
  measures "d5" distance of L6.end L7.end
  measures "d6" diameter of A1
  measures "d11" diameter of A2
extrude "Extrude2" add sketch "Sketch1" against normal blind 25 contours L0 L1 L3 L6 L7 L9 A1 | L3 A0 L8 A1 | L1 A0 L8 A1 | A0 L8 A1 makes body 1
extrude "Extrude1" add sketch "Sketch1" along normal blind 2 separate body makes body 2
extrude "Extrude3" cut sketch "Sketch1" along normal blind 2 contours L2 L8 A2 | L2 A2 | L8 A2 bodies 2
sketch "Sketch2" plane through (0, 0, 0) normal (0, -1, 0) x (1, 0, 0)
  circle A0 centre (0, 35) radius 5.25
  line L0 (-36.5, 36.5) -> (-36.5, -36.5)
  line L1 (-36.5, -36.5) -> (36.5, -36.5)
  line L2 (36.5, -36.5) -> (36.5, 36.5)
  arc A1 (36.5, 36.5) -> (-36.5, 36.5) centre (0, 36.5) ccw
  line L3 (0, 0) -> (-1, 0)
  line L4 (-1, 0) -> (-1, 8)
  line L5 (-1, 8) -> (0, 8)
  line L6 (0, 8) -> (0, 0)
  circle A2 centre (0, 8) radius 4.5
  dimension "d14" = 1
  dimension "d15" = 8
  dimension "d16" = 9
  constraint horizontal L3
  constraint vertical L4
  constraint horizontal L5
  constraint vertical L6
  constraint coincident L3.start L6.end
  constraint coincident L5.end L6.start
  measures "d14" distance of L3.start L3.end
  measures "d15" distance of L3.start L5.end
  measures "d16" diameter of A2
extrude "Extrude4" add sketch "Sketch2" along normal blind 20 contours L4 L5 L6 A2 | L4 L5 L6 A2 bodies 2
sketch "Sketch3" plane through (0, -20, 0) normal (0, -1, 0) x (1, 0, 0)
  circle A0 centre (0, 8) radius 4.5
  circle A1 centre (0, 8) radius 2.6
  dimension "d19" = 5.2
  constraint concentric A0 A1
  measures "d19" diameter of A1
extrude "Extrude5" cut sketch "Sketch3" against normal blind 20 contours A1 bodies 2